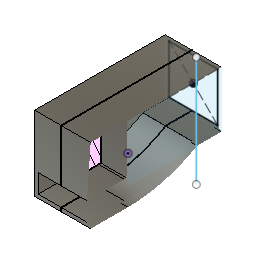
TAP-DIVERGE (Autodesk Fusion 360 design; units mm, degrees)
Autodesk Fusion 360 part; units mm, degrees
sketch "Sketch1" plane through (0, 0, 0) normal (0, 1, 0) x (1, 0, 0)
  line L0 (15, -15) -> (-15, -15)
  line L1 (-15, -15) -> (-15, 15)
  line L2 (-15, 15) -> (15, 15)
  line L3 (15, 15) -> (15, -15)
  line L4 (15, -15) -> (-15, 15) construction
  line L5 (-15, -15) -> (15, 15) construction
  dimension "d1" = 30
  dimension "d2" = 30
  constraint horizontal L0
  constraint perpendicular L0 L1
  constraint parallel L0 L2
  constraint parallel L1 L3
  constraint coincident L4 origin
  constraint coincident L5 origin
  measures "d1" distance of L1.end L2.end
  measures "d2" distance of L0.end L1.end
extrude "Extrude1" add sketch "Sketch1" along normal blind 50
sketch "Sketch3" plane through (15, 0, 0) normal (1, 0, 0) x (0, 1, 0)
  line L0 (0, 15) -> (0, -15)
  line L1 (0, -15) -> (50, -15)
  line L2 (50, -15) -> (50, 15)
  line L3 (50, 15) -> (0, 15)
  line L4 (36.5913, 26.2783) -> (36.5913, -32.7983)
  constraint vertical L4
sketch "Sketch4" plane through (15, 0, 0) normal (1, 0, 0) x (0, 1, 0)
sketch "Sketch5" plane through (15, 0, 0) normal (1, 0, 0) x (0, 1, 0)
  arc A0 (0, -25) -> (37, -15) centre (-0.3235, 49.6471) ccw
  line L0 (0, -25) -> (0, -15)
  line L1 (0, -15) -> (37, -15)
  constraint vertical L0
  constraint perpendicular L0 L1
extrude "Extrude3" add sketch "Sketch5" against normal blind 30
sketch "Sketch7" plane through (0, 50, 0) normal (0, 1, 0) x (-1, 0, 0)
  line L0 (-15, -15) -> (15, -15)
  line L1 (15, -15) -> (15, 15)
  line L2 (15, 15) -> (-15, 15)
  line L3 (-15, 15) -> (-15, -15)
  line L4 (13.05, -13.05) -> (-13.05, -13.05)
  line L5 (-13.05, -13.05) -> (-13.05, 13.05)
  line L6 (-13.05, 13.05) -> (13.05, 13.05)
  line L7 (13.05, 13.05) -> (13.05, -13.05)
  line L8 (13.05, -13.05) -> (-13.05, 13.05) construction
  line L9 (-13.05, -13.05) -> (13.05, 13.05) construction
  dimension "d18" = 26.1
  dimension "d19" = 26.1
  constraint horizontal L4
  constraint perpendicular L4 L5
  constraint parallel L4 L6
  constraint parallel L5 L7
  constraint coincident L8 origin
  constraint coincident L9 origin
  measures "d18" distance of L5.end L6.end
  measures "d19" distance of L4.end L5.end
extrude "Extrude4" cut sketch "Sketch7" against normal blind 48.8 contours L4 L5 L6 L7
sketch "Sketch8" plane through (0, 0, 0) normal (0, -1, 0) x (1, 0, 0)
  line L0 (15, -25) -> (15, 15)
  line L1 (15, 15) -> (-15, 15)
  line L2 (-15, 15) -> (-15, -25)
  line L3 (-15, -25) -> (15, -25)
  line L4 (-13.1, -13) -> (13, -13)
  line L5 (13, -13) -> (13, -23)
  line L6 (13, -23) -> (-13.1, -23)
  line L7 (-13.1, -23) -> (-13.1, -13)
  dimension "d28" = 10
  dimension "d29" = 26.1
  constraint horizontal L4
  constraint perpendicular L4 L5
  constraint perpendicular L5 L6
  constraint perpendicular L4 L7
  measures "d28" distance of L4.end L5.end
  measures "d29" distance of L5.end L6.end
sweep "Sweep2" cut profiles "Sketch8" along 1 edges at (15, 19.1527, -22.4152) section 1 contours L4 L5 L6 L7
sketch "Sketch9" plane through (0, 0, 0) normal (0, -1, 0) x (1, 0, 0)
  line L0 (13, -13) -> (13, -23)
  line L1 (13, -23) -> (-13.1, -23)
  line L2 (-13.1, -23) -> (-13.1, -13)
  line L3 (-13.1, -13) -> (13, -13)
  line L4 (15, -25) -> (15, 15)
  line L5 (15, 15) -> (-15, 15)
  line L6 (-15, 15) -> (-15, -25)
  line L7 (-15, -25) -> (15, -25)
  line L8 (-15, 15) -> (-15, -25)
  line L9 (15, -25) -> (15, 15)
  line L10 (-13.1, -13) -> (13, -13)
  line L11 (13, -13) -> (13, -23)
  line L12 (13, -23) -> (-13.1, -23)
  line L13 (-13.1, -23) -> (-13.1, -13)
  constraint coincident L5.end L6.start
  constraint coincident L6.end L7.start
  constraint coincident L4.start L7.end
  constraint coincident L4.end L5.start
  constraint horizontal L10
  constraint vertical L11
  constraint horizontal L12
  constraint vertical L13
  constraint coincident L0.end L1.start
  constraint coincident L2.end L3.start
extrude "Extrude5" add sketch "Sketch9" along normal blind 20
